Autodesk Fusion 360 part; units mm, degrees
(part 4 of 5)
sketch "Sketch4" plane through (0, 0, 0) normal (0, 0, -1) x (-1, 0, 0)
  arc A0 (-100, 198) -> (-100, 202) centre (-100, 200) ccw
  line L0 (-100, 198) -> (-100, 162)
  arc A1 (-100, 158) -> (-100, 162) centre (-100, 160) ccw
  line L1 (-100, 158) -> (-100, 122)
  arc A2 (-100, 118) -> (-100, 122) centre (-100, 120) ccw
  line L2 (-100, 118) -> (-100, 82)
  arc A3 (-100, 78) -> (-100, 82) centre (-100, 80) ccw
  line L3 (-100, 78) -> (-100, 42)
  arc A4 (-100, 38) -> (-100, 42) centre (-100, 40) ccw
  line L4 (-100, 38) -> (-100, 2)
  arc A5 (-100, -2) -> (-100, 2) centre (-100, 0) ccw
  line L5 (-100, -2) -> (-100, -38)
  arc A6 (-100, -42) -> (-100, -38) centre (-100, -40) ccw
  line L6 (-100, -42) -> (-100, -78)
  arc A7 (-100, -82) -> (-100, -78) centre (-100, -80) ccw
  line L7 (-100, -82) -> (-100, -118)
  arc A8 (-100, -122) -> (-100, -118) centre (-100, -120) ccw
  line L8 (-100, -122) -> (-100, -158)
  arc A9 (-100, -162) -> (-100, -158) centre (-100, -160) ccw
  line L9 (-100, -162) -> (-100, -198)
  arc A10 (-100, -202) -> (-100, -198) centre (-100, -200) ccw
  line L10 (-100, -202) -> (-100, -220)
  line L11 (-100, -220) -> (100, -220)
  line L12 (100, -220) -> (100, 220)
  line L13 (100, 220) -> (-100, 220)
  line L14 (-100, 220) -> (-100, 202)
  line L15 (38.5, 121.5) -> (21.5, 121.5)
  line L16 (21.5, 121.5) -> (21.5, 138.5)
  line L17 (21.5, 138.5) -> (38.5, 138.5)
  line L18 (38.5, 138.5) -> (38.5, 121.5)
  line L19 (18.5, 121.5) -> (1.5, 121.5)
  line L20 (1.5, 121.5) -> (1.5, 138.5)
  line L21 (1.5, 138.5) -> (18.5, 138.5)
  line L22 (18.5, 138.5) -> (18.5, 121.5)
  line L23 (-1.5, 121.5) -> (-18.5, 121.5)
  line L24 (-18.5, 121.5) -> (-18.5, 138.5)
  line L25 (-18.5, 138.5) -> (-1.5, 138.5)
  line L26 (-1.5, 138.5) -> (-1.5, 121.5)
  line L27 (-21.5, 121.5) -> (-38.5, 121.5)
  line L28 (-38.5, 121.5) -> (-38.5, 138.5)
  line L29 (-38.5, 138.5) -> (-21.5, 138.5)
  line L30 (-21.5, 138.5) -> (-21.5, 121.5)
  line L31 (-41.5, 121.5) -> (-58.5, 121.5)
  line L32 (-58.5, 121.5) -> (-58.5, 138.5)
  line L33 (-58.5, 138.5) -> (-41.5, 138.5)
  line L34 (-41.5, 138.5) -> (-41.5, 121.5)
  line L35 (-61.5, 121.5) -> (-78.5, 121.5)
  line L36 (-78.5, 121.5) -> (-78.5, 138.5)
  line L37 (-78.5, 138.5) -> (-61.5, 138.5)
  line L38 (-61.5, 138.5) -> (-61.5, 121.5)
  line L39 (-81.5, 121.5) -> (-98.5, 121.5)
  line L40 (-98.5, 121.5) -> (-98.5, 138.5)
  line L41 (-98.5, 138.5) -> (-81.5, 138.5)
  line L42 (-81.5, 138.5) -> (-81.5, 121.5)
  line L43 (98.5, 141.5) -> (81.5, 141.5)
  line L44 (81.5, 141.5) -> (81.5, 158.5)
  line L45 (81.5, 158.5) -> (98.5, 158.5)
  line L46 (98.5, 158.5) -> (98.5, 141.5)
  line L47 (78.5, 141.5) -> (61.5, 141.5)
  line L48 (61.5, 141.5) -> (61.5, 158.5)
  line L49 (61.5, 158.5) -> (78.5, 158.5)
  line L50 (78.5, 158.5) -> (78.5, 141.5)
  line L51 (58.5, 141.5) -> (41.5, 141.5)
  line L52 (41.5, 141.5) -> (41.5, 158.5)
  line L53 (41.5, 158.5) -> (58.5, 158.5)
  line L54 (58.5, 158.5) -> (58.5, 141.5)
  line L55 (38.5, 141.5) -> (21.5, 141.5)
  line L56 (21.5, 141.5) -> (21.5, 158.5)
  line L57 (21.5, 158.5) -> (38.5, 158.5)
  line L58 (38.5, 158.5) -> (38.5, 141.5)
  line L59 (18.5, 141.5) -> (1.5, 141.5)
  line L60 (1.5, 141.5) -> (1.5, 158.5)
  line L61 (1.5, 158.5) -> (18.5, 158.5)
  line L62 (18.5, 158.5) -> (18.5, 141.5)
  line L63 (-1.5, 141.5) -> (-18.5, 141.5)
  line L64 (-18.5, 141.5) -> (-18.5, 158.5)
  line L65 (-18.5, 158.5) -> (-1.5, 158.5)
  line L66 (-1.5, 158.5) -> (-1.5, 141.5)
  line L67 (-21.5, 141.5) -> (-38.5, 141.5)
  line L68 (-38.5, 141.5) -> (-38.5, 158.5)
  line L69 (-38.5, 158.5) -> (-21.5, 158.5)
  line L70 (-21.5, 158.5) -> (-21.5, 141.5)
  line L71 (-41.5, 141.5) -> (-58.5, 141.5)
  line L72 (-58.5, 141.5) -> (-58.5, 158.5)
  line L73 (-58.5, 158.5) -> (-41.5, 158.5)
  line L74 (-41.5, 158.5) -> (-41.5, 141.5)
  line L75 (-61.5, 141.5) -> (-78.5, 141.5)
  line L76 (-78.5, 141.5) -> (-78.5, 158.5)
  line L77 (-78.5, 158.5) -> (-61.5, 158.5)
  line L78 (-61.5, 158.5) -> (-61.5, 141.5)
  line L79 (-81.5, 141.5) -> (-98.5, 141.5)
  line L80 (-98.5, 141.5) -> (-98.5, 158.5)
  line L81 (-98.5, 158.5) -> (-81.5, 158.5)
  line L82 (-81.5, 158.5) -> (-81.5, 141.5)
  line L83 (98.5, 161.5) -> (81.5, 161.5)
  line L84 (81.5, 161.5) -> (81.5, 178.5)
  line L85 (81.5, 178.5) -> (98.5, 178.5)
  line L86 (98.5, 178.5) -> (98.5, 161.5)
  line L87 (78.5, 161.5) -> (61.5, 161.5)
  line L88 (61.5, 161.5) -> (61.5, 178.5)
  line L89 (61.5, 178.5) -> (78.5, 178.5)
  line L90 (78.5, 178.5) -> (78.5, 161.5)
  line L91 (58.5, 161.5) -> (41.5, 161.5)
  line L92 (41.5, 161.5) -> (41.5, 178.5)
  line L93 (41.5, 178.5) -> (58.5, 178.5)
  line L94 (58.5, 178.5) -> (58.5, 161.5)
  line L95 (58.5, 121.5) -> (41.5, 121.5)
  line L96 (41.5, 121.5) -> (41.5, 138.5)
  line L97 (41.5, 138.5) -> (58.5, 138.5)
  line L98 (58.5, 138.5) -> (58.5, 121.5)
  line L99 (98.5, -98.5) -> (81.5, -98.5)
  line L100 (81.5, -98.5) -> (81.5, -81.5)
  line L101 (81.5, -81.5) -> (98.5, -81.5)
  line L102 (98.5, -81.5) -> (98.5, -98.5)
  line L103 (-1.5, -58.5) -> (-18.5, -58.5)
  line L104 (-18.5, -58.5) -> (-18.5, -41.5)
  line L105 (-18.5, -41.5) -> (-1.5, -41.5)
  line L106 (-1.5, -41.5) -> (-1.5, -58.5)
  line L107 (-81.5, -118.5) -> (-98.5, -118.5)
  line L108 (-98.5, -118.5) -> (-98.5, -101.5)
  line L109 (-98.5, -101.5) -> (-81.5, -101.5)
  line L110 (-81.5, -101.5) -> (-81.5, -118.5)
  line L111 (-61.5, -118.5) -> (-78.5, -118.5)
  line L112 (-78.5, -118.5) -> (-78.5, -101.5)
  line L113 (-78.5, -101.5) -> (-61.5, -101.5)
  line L114 (-61.5, -101.5) -> (-61.5, -118.5)
  line L115 (-41.5, -118.5) -> (-58.5, -118.5)
  line L116 (-58.5, -118.5) -> (-58.5, -101.5)
  line L117 (-58.5, -101.5) -> (-41.5, -101.5)
  line L118 (-41.5, -101.5) -> (-41.5, -118.5)
  line L119 (-21.5, -118.5) -> (-38.5, -118.5)
  line L120 (-38.5, -118.5) -> (-38.5, -101.5)
  line L121 (-38.5, -101.5) -> (-21.5, -101.5)
  line L122 (-21.5, -101.5) -> (-21.5, -118.5)
  line L123 (-1.5, -118.5) -> (-18.5, -118.5)
  line L124 (-18.5, -118.5) -> (-18.5, -101.5)
  line L125 (-18.5, -101.5) -> (-1.5, -101.5)
  line L126 (-1.5, -101.5) -> (-1.5, -118.5)
  line L127 (18.5, -118.5) -> (1.5, -118.5)
  line L128 (1.5, -118.5) -> (1.5, -101.5)
  line L129 (1.5, -101.5) -> (18.5, -101.5)
  line L130 (18.5, -101.5) -> (18.5, -118.5)
  line L131 (38.5, -118.5) -> (21.5, -118.5)
  line L132 (21.5, -118.5) -> (21.5, -101.5)
  line L133 (21.5, -101.5) -> (38.5, -101.5)
  line L134 (38.5, -101.5) -> (38.5, -118.5)
  line L135 (58.5, -118.5) -> (41.5, -118.5)
  line L136 (41.5, -118.5) -> (41.5, -101.5)
  line L137 (41.5, -101.5) -> (58.5, -101.5)
  line L138 (58.5, -101.5) -> (58.5, -118.5)
  line L139 (78.5, -118.5) -> (61.5, -118.5)
  line L140 (61.5, -118.5) -> (61.5, -101.5)
  line L141 (61.5, -101.5) -> (78.5, -101.5)
  line L142 (78.5, -101.5) -> (78.5, -118.5)
  line L143 (98.5, -118.5) -> (81.5, -118.5)
  line L144 (81.5, -118.5) -> (81.5, -101.5)
  line L145 (81.5, -101.5) -> (98.5, -101.5)
  line L146 (98.5, -101.5) -> (98.5, -118.5)
  line L147 (-81.5, -138.5) -> (-98.5, -138.5)
  line L148 (-98.5, -138.5) -> (-98.5, -121.5)
  line L149 (-98.5, -121.5) -> (-81.5, -121.5)
  line L150 (-81.5, -121.5) -> (-81.5, -138.5)
  line L151 (-61.5, -138.5) -> (-78.5, -138.5)
  line L152 (-78.5, -138.5) -> (-78.5, -121.5)
  line L153 (-78.5, -121.5) -> (-61.5, -121.5)
  line L154 (-61.5, -121.5) -> (-61.5, -138.5)
  line L155 (-41.5, -138.5) -> (-58.5, -138.5)
  line L156 (-58.5, -138.5) -> (-58.5, -121.5)
  line L157 (-58.5, -121.5) -> (-41.5, -121.5)
  line L158 (-41.5, -121.5) -> (-41.5, -138.5)
  line L159 (-21.5, -138.5) -> (-38.5, -138.5)
  line L160 (-38.5, -138.5) -> (-38.5, -121.5)
  line L161 (-38.5, -121.5) -> (-21.5, -121.5)
  line L162 (-21.5, -121.5) -> (-21.5, -138.5)
  line L163 (-1.5, -138.5) -> (-18.5, -138.5)
  line L164 (-18.5, -138.5) -> (-18.5, -121.5)
  line L165 (-18.5, -121.5) -> (-1.5, -121.5)
  line L166 (-1.5, -121.5) -> (-1.5, -138.5)
  line L167 (18.5, -138.5) -> (1.5, -138.5)
  line L168 (1.5, -138.5) -> (1.5, -121.5)
  line L169 (1.5, -121.5) -> (18.5, -121.5)
  line L170 (18.5, -121.5) -> (18.5, -138.5)
  line L171 (38.5, -138.5) -> (21.5, -138.5)
  line L172 (21.5, -138.5) -> (21.5, -121.5)
  line L173 (21.5, -121.5) -> (38.5, -121.5)
  line L174 (38.5, -121.5) -> (38.5, -138.5)
  line L175 (58.5, -138.5) -> (41.5, -138.5)
  line L176 (41.5, -138.5) -> (41.5, -121.5)
  line L177 (41.5, -121.5) -> (58.5, -121.5)
  line L178 (58.5, -121.5) -> (58.5, -138.5)
  line L179 (78.5, -138.5) -> (61.5, -138.5)
  line L180 (61.5, -138.5) -> (61.5, -121.5)
  line L181 (61.5, -121.5) -> (78.5, -121.5)
  line L182 (78.5, -121.5) -> (78.5, -138.5)
  line L183 (98.5, -138.5) -> (81.5, -138.5)
  line L184 (81.5, -138.5) -> (81.5, -121.5)
  line L185 (81.5, -121.5) -> (98.5, -121.5)
  line L186 (98.5, -121.5) -> (98.5, -138.5)
  line L187 (-81.5, -158.5) -> (-98.5, -158.5)
  line L188 (-98.5, -158.5) -> (-98.5, -141.5)
  line L189 (-98.5, -141.5) -> (-81.5, -141.5)
  line L190 (-81.5, -141.5) -> (-81.5, -158.5)
  line L191 (-61.5, -158.5) -> (-78.5, -158.5)
  line L192 (-78.5, -158.5) -> (-78.5, -141.5)
  line L193 (-78.5, -141.5) -> (-61.5, -141.5)
  line L194 (-61.5, -141.5) -> (-61.5, -158.5)
  line L195 (-41.5, -158.5) -> (-58.5, -158.5)
  line L196 (-58.5, -158.5) -> (-58.5, -141.5)
  line L197 (-58.5, -141.5) -> (-41.5, -141.5)
  line L198 (-41.5, -141.5) -> (-41.5, -158.5)
  line L199 (-21.5, -158.5) -> (-38.5, -158.5)
  line L200 (-38.5, -158.5) -> (-38.5, -141.5)
  line L201 (-38.5, -141.5) -> (-21.5, -141.5)
  line L202 (-21.5, -141.5) -> (-21.5, -158.5)
  line L203 (-1.5, -158.5) -> (-18.5, -158.5)
  line L204 (-18.5, -158.5) -> (-18.5, -141.5)
  line L205 (-18.5, -141.5) -> (-1.5, -141.5)
  line L206 (-1.5, -141.5) -> (-1.5, -158.5)
  line L207 (18.5, -158.5) -> (1.5, -158.5)
  line L208 (1.5, -158.5) -> (1.5, -141.5)
  line L209 (1.5, -141.5) -> (18.5, -141.5)
  line L210 (18.5, -141.5) -> (18.5, -158.5)
  line L211 (38.5, -158.5) -> (21.5, -158.5)
  line L212 (21.5, -158.5) -> (21.5, -141.5)
  line L213 (21.5, -141.5) -> (38.5, -141.5)
  line L214 (38.5, -141.5) -> (38.5, -158.5)
  line L215 (58.5, -158.5) -> (41.5, -158.5)
  line L216 (41.5, -158.5) -> (41.5, -141.5)
  line L217 (41.5, -141.5) -> (58.5, -141.5)
  line L218 (58.5, -141.5) -> (58.5, -158.5)
  line L219 (-41.5, -58.5) -> (-58.5, -58.5)
  line L220 (-58.5, -58.5) -> (-58.5, -41.5)
  line L221 (-58.5, -41.5) -> (-41.5, -41.5)
  line L222 (-41.5, -41.5) -> (-41.5, -58.5)
  line L223 (98.5, -201.5) -> (98.5, -218.5)
  line L224 (98.5, -218.5) -> (81.5, -218.5)
  line L225 (81.5, -218.5) -> (81.5, -201.5)
  line L226 (81.5, -201.5) -> (98.5, -201.5)
  line L227 (78.5, -218.5) -> (61.5, -218.5)
  line L228 (61.5, -218.5) -> (61.5, -201.5)
  line L229 (61.5, -201.5) -> (78.5, -201.5)
  line L230 (78.5, -201.5) -> (78.5, -218.5)
  line L231 (58.5, -218.5) -> (41.5, -218.5)
  line L232 (41.5, -218.5) -> (41.5, -201.5)
  line L233 (41.5, -201.5) -> (58.5, -201.5)
  line L234 (58.5, -201.5) -> (58.5, -218.5)
  line L235 (38.5, -218.5) -> (21.5, -218.5)
  line L236 (21.5, -218.5) -> (21.5, -201.5)
  line L237 (21.5, -201.5) -> (38.5, -201.5)
  line L238 (38.5, -201.5) -> (38.5, -218.5)
  line L239 (18.5, -218.5) -> (1.5, -218.5)
  line L240 (1.5, -218.5) -> (1.5, -201.5)
  line L241 (1.5, -201.5) -> (18.5, -201.5)
  line L242 (18.5, -201.5) -> (18.5, -218.5)
  line L243 (-1.5, -218.5) -> (-18.5, -218.5)
  line L244 (-18.5, -218.5) -> (-18.5, -201.5)
  line L245 (-18.5, -201.5) -> (-1.5, -201.5)
  line L246 (-1.5, -201.5) -> (-1.5, -218.5)
  line L247 (-21.5, -218.5) -> (-38.5, -218.5)
  line L248 (-38.5, -218.5) -> (-38.5, -201.5)
  line L249 (-38.5, -201.5) -> (-21.5, -201.5)
  line L250 (-21.5, -201.5) -> (-21.5, -218.5)
  line L251 (-41.5, -218.5) -> (-58.5, -218.5)
  line L252 (-58.5, -218.5) -> (-58.5, -201.5)
  line L253 (-58.5, -201.5) -> (-41.5, -201.5)
  line L254 (-41.5, -201.5) -> (-41.5, -218.5)
  line L255 (-61.5, -218.5) -> (-78.5, -218.5)
  line L256 (-78.5, -218.5) -> (-78.5, -201.5)
  line L257 (-78.5, -201.5) -> (-61.5, -201.5)
  line L258 (-61.5, -201.5) -> (-61.5, -218.5)
  line L259 (-81.5, -218.5) -> (-98.5, -218.5)
  line L260 (-98.5, -218.5) -> (-98.5, -201.5)
  line L261 (-98.5, -201.5) -> (-81.5, -201.5)
  line L262 (-81.5, -201.5) -> (-81.5, -218.5)
  line L263 (98.5, -198.5) -> (81.5, -198.5)
  line L264 (81.5, -198.5) -> (81.5, -181.5)
  line L265 (81.5, -181.5) -> (98.5, -181.5)
  line L266 (98.5, -181.5) -> (98.5, -198.5)
  line L267 (78.5, -198.5) -> (61.5, -198.5)
  line L268 (61.5, -198.5) -> (61.5, -181.5)
  line L269 (61.5, -181.5) -> (78.5, -181.5)
  line L270 (78.5, -181.5) -> (78.5, -198.5)
  line L271 (58.5, -198.5) -> (41.5, -198.5)
  line L272 (41.5, -198.5) -> (41.5, -181.5)
  line L273 (41.5, -181.5) -> (58.5, -181.5)
  line L274 (58.5, -181.5) -> (58.5, -198.5)
  line L275 (38.5, -198.5) -> (21.5, -198.5)
  line L276 (21.5, -198.5) -> (21.5, -181.5)
  line L277 (21.5, -181.5) -> (38.5, -181.5)
  line L278 (38.5, -181.5) -> (38.5, -198.5)
  line L279 (18.5, -198.5) -> (1.5, -198.5)
  line L280 (1.5, -198.5) -> (1.5, -181.5)
  line L281 (1.5, -181.5) -> (18.5, -181.5)
  line L282 (18.5, -181.5) -> (18.5, -198.5)
  line L283 (-1.5, -198.5) -> (-18.5, -198.5)
  line L284 (-18.5, -198.5) -> (-18.5, -181.5)
  line L285 (-18.5, -181.5) -> (-1.5, -181.5)
  line L286 (-1.5, -181.5) -> (-1.5, -198.5)
  line L287 (-21.5, -198.5) -> (-38.5, -198.5)
  line L288 (-38.5, -198.5) -> (-38.5, -181.5)
  line L289 (-38.5, -181.5) -> (-21.5, -181.5)
  line L290 (-21.5, -181.5) -> (-21.5, -198.5)
  line L291 (-41.5, -198.5) -> (-58.5, -198.5)
  line L292 (-58.5, -198.5) -> (-58.5, -181.5)
  line L293 (-58.5, -181.5) -> (-41.5, -181.5)
  line L294 (-41.5, -181.5) -> (-41.5, -198.5)
  line L295 (-61.5, -198.5) -> (-78.5, -198.5)
  line L296 (-78.5, -198.5) -> (-78.5, -181.5)
  line L297 (-78.5, -181.5) -> (-61.5, -181.5)
  line L298 (-61.5, -181.5) -> (-61.5, -198.5)
  line L299 (-81.5, -198.5) -> (-98.5, -198.5)
  line L300 (-98.5, -198.5) -> (-98.5, -181.5)
  line L301 (-98.5, -181.5) -> (-81.5, -181.5)
  line L302 (-81.5, -181.5) -> (-81.5, -198.5)
  line L303 (98.5, -178.5) -> (81.5, -178.5)
  line L304 (81.5, -178.5) -> (81.5, -161.5)
  line L305 (81.5, -161.5) -> (98.5, -161.5)
  line L306 (98.5, -161.5) -> (98.5, -178.5)
  line L307 (78.5, -178.5) -> (61.5, -178.5)
  line L308 (61.5, -178.5) -> (61.5, -161.5)
  line L309 (61.5, -161.5) -> (78.5, -161.5)
  line L310 (78.5, -161.5) -> (78.5, -178.5)
  line L311 (58.5, -178.5) -> (41.5, -178.5)
  line L312 (41.5, -178.5) -> (41.5, -161.5)
  line L313 (41.5, -161.5) -> (58.5, -161.5)
  line L314 (58.5, -161.5) -> (58.5, -178.5)
  line L315 (38.5, -178.5) -> (21.5, -178.5)
  line L316 (21.5, -178.5) -> (21.5, -161.5)
  line L317 (21.5, -161.5) -> (38.5, -161.5)
  line L318 (38.5, -161.5) -> (38.5, -178.5)
  line L319 (18.5, -178.5) -> (1.5, -178.5)
  line L320 (1.5, -178.5) -> (1.5, -161.5)
  line L321 (1.5, -161.5) -> (18.5, -161.5)
  line L322 (18.5, -161.5) -> (18.5, -178.5)
  line L323 (-1.5, -178.5) -> (-18.5, -178.5)
  line L324 (-18.5, -178.5) -> (-18.5, -161.5)
  line L325 (-18.5, -161.5) -> (-1.5, -161.5)
  line L326 (-1.5, -161.5) -> (-1.5, -178.5)
  line L327 (98.5, -158.5) -> (81.5, -158.5)
  line L328 (81.5, -158.5) -> (81.5, -141.5)
  line L329 (81.5, -141.5) -> (98.5, -141.5)
  line L330 (98.5, -141.5) -> (98.5, -158.5)
  line L331 (78.5, -158.5) -> (61.5, -158.5)
  line L332 (61.5, -158.5) -> (61.5, -141.5)
  line L333 (61.5, -141.5) -> (78.5, -141.5)
  line L334 (78.5, -141.5) -> (78.5, -158.5)
  line L335 (-81.5, -178.5) -> (-98.5, -178.5)
  line L336 (-98.5, -178.5) -> (-98.5, -161.5)
  line L337 (-98.5, -161.5) -> (-81.5, -161.5)
  line L338 (-81.5, -161.5) -> (-81.5, -178.5)
  line L339 (-61.5, -178.5) -> (-78.5, -178.5)
  line L340 (-78.5, -178.5) -> (-78.5, -161.5)
  line L341 (-78.5, -161.5) -> (-61.5, -161.5)
  line L342 (-61.5, -161.5) -> (-61.5, -178.5)
  line L343 (-41.5, -178.5) -> (-58.5, -178.5)
  line L344 (-58.5, -178.5) -> (-58.5, -161.5)
  line L345 (-58.5, -161.5) -> (-41.5, -161.5)
  line L346 (-41.5, -161.5) -> (-41.5, -178.5)
  line L347 (-21.5, -178.5) -> (-38.5, -178.5)
  line L348 (-38.5, -178.5) -> (-38.5, -161.5)
  line L349 (-38.5, -161.5) -> (-21.5, -161.5)
  line L350 (-21.5, -161.5) -> (-21.5, -178.5)
  line L351 (38.5, 161.5) -> (21.5, 161.5)
  line L352 (21.5, 161.5) -> (21.5, 178.5)
  line L353 (21.5, 178.5) -> (38.5, 178.5)
  line L354 (38.5, 178.5) -> (38.5, 161.5)
  line L355 (78.5, -98.5) -> (61.5, -98.5)
  line L356 (61.5, -98.5) -> (61.5, -81.5)
  line L357 (61.5, -81.5) -> (78.5, -81.5)
  line L358 (78.5, -81.5) -> (78.5, -98.5)
  line L359 (98.5, 121.5) -> (81.5, 121.5)
  line L360 (81.5, 121.5) -> (81.5, 138.5)
  line L361 (81.5, 138.5) -> (98.5, 138.5)
  line L362 (98.5, 138.5) -> (98.5, 121.5)
  line L363 (-81.5, 101.5) -> (-98.5, 101.5)
  line L364 (-98.5, 101.5) -> (-98.5, 118.5)
  line L365 (-98.5, 118.5) -> (-81.5, 118.5)
  line L366 (-81.5, 118.5) -> (-81.5, 101.5)
  line L367 (-61.5, 101.5) -> (-78.5, 101.5)
  line L368 (-78.5, 101.5) -> (-78.5, 118.5)
  line L369 (-78.5, 118.5) -> (-61.5, 118.5)
  line L370 (-61.5, 118.5) -> (-61.5, 101.5)
  line L371 (-41.5, 101.5) -> (-58.5, 101.5)
  line L372 (-58.5, 101.5) -> (-58.5, 118.5)
  line L373 (-58.5, 118.5) -> (-41.5, 118.5)
  line L374 (-41.5, 118.5) -> (-41.5, 101.5)
  line L375 (-21.5, 101.5) -> (-38.5, 101.5)
  line L376 (-38.5, 101.5) -> (-38.5, 118.5)
  line L377 (-38.5, 118.5) -> (-21.5, 118.5)
  line L378 (-21.5, 118.5) -> (-21.5, 101.5)
  line L379 (-1.5, 101.5) -> (-18.5, 101.5)
  line L380 (-18.5, 101.5) -> (-18.5, 118.5)
  line L381 (-18.5, 118.5) -> (-1.5, 118.5)
  line L382 (-1.5, 118.5) -> (-1.5, 101.5)
  line L383 (18.5, 101.5) -> (1.5, 101.5)
  line L384 (1.5, 101.5) -> (1.5, 118.5)
  line L385 (1.5, 118.5) -> (18.5, 118.5)
  line L386 (18.5, 118.5) -> (18.5, 101.5)
  line L387 (38.5, 101.5) -> (21.5, 101.5)
  line L388 (21.5, 101.5) -> (21.5, 118.5)
  line L389 (21.5, 118.5) -> (38.5, 118.5)
  line L390 (38.5, 118.5) -> (38.5, 101.5)
  line L391 (58.5, 101.5) -> (41.5, 101.5)
  line L392 (41.5, 101.5) -> (41.5, 118.5)
  line L393 (41.5, 118.5) -> (58.5, 118.5)
  line L394 (58.5, 118.5) -> (58.5, 101.5)
  line L395 (78.5, 101.5) -> (61.5, 101.5)
  line L396 (61.5, 101.5) -> (61.5, 118.5)
  line L397 (61.5, 118.5) -> (78.5, 118.5)
  line L398 (78.5, 118.5) -> (78.5, 101.5)
  line L399 (98.5, 101.5) -> (81.5, 101.5)
  line L400 (81.5, 101.5) -> (81.5, 118.5)
  line L401 (81.5, 118.5) -> (98.5, 118.5)
  line L402 (98.5, 118.5) -> (98.5, 101.5)
  line L403 (-81.5, 81.5) -> (-98.5, 81.5)
  line L404 (-98.5, 81.5) -> (-98.5, 98.5)
  line L405 (-98.5, 98.5) -> (-81.5, 98.5)
  line L406 (-81.5, 98.5) -> (-81.5, 81.5)
  line L407 (-61.5, 81.5) -> (-78.5, 81.5)
  line L408 (-78.5, 81.5) -> (-78.5, 98.5)
  line L409 (-78.5, 98.5) -> (-61.5, 98.5)
  line L410 (-61.5, 98.5) -> (-61.5, 81.5)
  line L411 (-41.5, 81.5) -> (-58.5, 81.5)
  line L412 (-58.5, 81.5) -> (-58.5, 98.5)
  line L413 (-58.5, 98.5) -> (-41.5, 98.5)
  line L414 (-41.5, 98.5) -> (-41.5, 81.5)
  line L415 (-21.5, 81.5) -> (-38.5, 81.5)
  line L416 (-38.5, 81.5) -> (-38.5, 98.5)
  line L417 (-38.5, 98.5) -> (-21.5, 98.5)
  line L418 (-21.5, 98.5) -> (-21.5, 81.5)
  line L419 (-1.5, 81.5) -> (-18.5, 81.5)
  line L420 (-18.5, 81.5) -> (-18.5, 98.5)
  line L421 (-18.5, 98.5) -> (-1.5, 98.5)
  line L422 (-1.5, 98.5) -> (-1.5, 81.5)
  line L423 (18.5, 81.5) -> (1.5, 81.5)
  line L424 (1.5, 81.5) -> (1.5, 98.5)
  line L425 (1.5, 98.5) -> (18.5, 98.5)
  line L426 (18.5, 98.5) -> (18.5, 81.5)
  line L427 (38.5, 81.5) -> (21.5, 81.5)
  line L428 (21.5, 81.5) -> (21.5, 98.5)
  line L429 (21.5, 98.5) -> (38.5, 98.5)
  line L430 (38.5, 98.5) -> (38.5, 81.5)
  line L431 (58.5, 81.5) -> (41.5, 81.5)
  line L432 (41.5, 81.5) -> (41.5, 98.5)
  line L433 (41.5, 98.5) -> (58.5, 98.5)
  line L434 (58.5, 98.5) -> (58.5, 81.5)
  line L435 (78.5, 81.5) -> (61.5, 81.5)
  line L436 (61.5, 81.5) -> (61.5, 98.5)
  line L437 (61.5, 98.5) -> (78.5, 98.5)
  line L438 (78.5, 98.5) -> (78.5, 81.5)
  line L439 (98.5, 81.5) -> (81.5, 81.5)
  line L440 (81.5, 81.5) -> (81.5, 98.5)
  line L441 (81.5, 98.5) -> (98.5, 98.5)
  line L442 (98.5, 98.5) -> (98.5, 81.5)
  line L443 (-81.5, 61.5) -> (-98.5, 61.5)
  line L444 (-98.5, 61.5) -> (-98.5, 78.5)
  line L445 (-98.5, 78.5) -> (-81.5, 78.5)
  line L446 (-81.5, 78.5) -> (-81.5, 61.5)
  line L447 (-61.5, 61.5) -> (-78.5, 61.5)
  line L448 (-78.5, 61.5) -> (-78.5, 78.5)
  line L449 (-78.5, 78.5) -> (-61.5, 78.5)
  line L450 (-61.5, 78.5) -> (-61.5, 61.5)
  line L451 (-41.5, 61.5) -> (-58.5, 61.5)
  line L452 (-58.5, 61.5) -> (-58.5, 78.5)
  line L453 (-58.5, 78.5) -> (-41.5, 78.5)
  line L454 (-41.5, 78.5) -> (-41.5, 61.5)
  line L455 (-21.5, 61.5) -> (-38.5, 61.5)
  line L456 (-38.5, 61.5) -> (-38.5, 78.5)
  line L457 (-38.5, 78.5) -> (-21.5, 78.5)
  line L458 (-21.5, 78.5) -> (-21.5, 61.5)
  line L459 (-1.5, 61.5) -> (-18.5, 61.5)
  line L460 (-18.5, 61.5) -> (-18.5, 78.5)
  line L461 (-18.5, 78.5) -> (-1.5, 78.5)
  line L462 (-1.5, 78.5) -> (-1.5, 61.5)
  line L463 (18.5, 61.5) -> (1.5, 61.5)
  line L464 (1.5, 61.5) -> (1.5, 78.5)
  line L465 (1.5, 78.5) -> (18.5, 78.5)
  line L466 (18.5, 78.5) -> (18.5, 61.5)
  line L467 (38.5, 61.5) -> (21.5, 61.5)
  line L468 (21.5, 61.5) -> (21.5, 78.5)
  line L469 (21.5, 78.5) -> (38.5, 78.5)
  line L470 (38.5, 78.5) -> (38.5, 61.5)
  line L471 (58.5, 61.5) -> (41.5, 61.5)
  line L472 (41.5, 61.5) -> (41.5, 78.5)
  line L473 (41.5, 78.5) -> (58.5, 78.5)
  line L474 (58.5, 78.5) -> (58.5, 61.5)
  line L475 (78.5, 61.5) -> (61.5, 61.5)
  line L476 (61.5, 61.5) -> (61.5, 78.5)
  line L477 (61.5, 78.5) -> (78.5, 78.5)
  line L478 (78.5, 78.5) -> (78.5, 61.5)
  line L479 (98.5, 61.5) -> (81.5, 61.5)
  line L480 (81.5, 61.5) -> (81.5, 78.5)
  line L481 (81.5, 78.5) -> (98.5, 78.5)
  line L482 (98.5, 78.5) -> (98.5, 61.5)
  line L483 (-81.5, 41.5) -> (-98.5, 41.5)
  line L484 (-98.5, 41.5) -> (-98.5, 58.5)
  line L485 (-98.5, 58.5) -> (-81.5, 58.5)
  line L486 (-81.5, 58.5) -> (-81.5, 41.5)
  line L487 (-61.5, 41.5) -> (-78.5, 41.5)
  line L488 (-78.5, 41.5) -> (-78.5, 58.5)
  line L489 (-78.5, 58.5) -> (-61.5, 58.5)
  line L490 (-61.5, 58.5) -> (-61.5, 41.5)
  line L491 (-41.5, 41.5) -> (-58.5, 41.5)
  line L492 (-58.5, 41.5) -> (-58.5, 58.5)
  line L493 (-58.5, 58.5) -> (-41.5, 58.5)
  line L494 (-41.5, 58.5) -> (-41.5, 41.5)
  line L495 (-21.5, 41.5) -> (-38.5, 41.5)
  line L496 (-38.5, 41.5) -> (-38.5, 58.5)
  line L497 (-38.5, 58.5) -> (-21.5, 58.5)
  line L498 (-21.5, 58.5) -> (-21.5, 41.5)
  line L499 (-1.5, 41.5) -> (-18.5, 41.5)
  line L500 (-18.5, 41.5) -> (-18.5, 58.5)
  line L501 (-18.5, 58.5) -> (-1.5, 58.5)
  line L502 (-1.5, 58.5) -> (-1.5, 41.5)
  line L503 (18.5, 41.5) -> (1.5, 41.5)
  line L504 (1.5, 41.5) -> (1.5, 58.5)
  line L505 (1.5, 58.5) -> (18.5, 58.5)
  line L506 (18.5, 58.5) -> (18.5, 41.5)
  line L507 (38.5, 41.5) -> (21.5, 41.5)
  line L508 (21.5, 41.5) -> (21.5, 58.5)
  line L509 (21.5, 58.5) -> (38.5, 58.5)
  line L510 (38.5, 58.5) -> (38.5, 41.5)
  line L511 (58.5, 41.5) -> (41.5, 41.5)
  line L512 (41.5, 41.5) -> (41.5, 58.5)
  line L513 (41.5, 58.5) -> (58.5, 58.5)
  line L514 (58.5, 58.5) -> (58.5, 41.5)
  line L515 (78.5, 41.5) -> (61.5, 41.5)
  line L516 (61.5, 41.5) -> (61.5, 58.5)
  line L517 (61.5, 58.5) -> (78.5, 58.5)
  line L518 (78.5, 58.5) -> (78.5, 41.5)
  line L519 (98.5, 41.5) -> (81.5, 41.5)
  line L520 (81.5, 41.5) -> (81.5, 58.5)
  line L521 (81.5, 58.5) -> (98.5, 58.5)
  line L522 (98.5, 58.5) -> (98.5, 41.5)
  line L523 (-81.5, 21.5) -> (-98.5, 21.5)
  line L524 (-98.5, 21.5) -> (-98.5, 38.5)
  line L525 (-98.5, 38.5) -> (-81.5, 38.5)
  line L526 (-81.5, 38.5) -> (-81.5, 21.5)
  line L527 (-61.5, 21.5) -> (-78.5, 21.5)
  line L528 (-78.5, 21.5) -> (-78.5, 38.5)
  line L529 (-78.5, 38.5) -> (-61.5, 38.5)
  line L530 (-61.5, 38.5) -> (-61.5, 21.5)
  line L531 (-41.5, 21.5) -> (-58.5, 21.5)
  line L532 (-58.5, 21.5) -> (-58.5, 38.5)
  line L533 (-58.5, 38.5) -> (-41.5, 38.5)
  line L534 (-41.5, 38.5) -> (-41.5, 21.5)
  line L535 (-21.5, 21.5) -> (-38.5, 21.5)
  line L536 (-38.5, 21.5) -> (-38.5, 38.5)
  line L537 (-38.5, 38.5) -> (-21.5, 38.5)
  line L538 (-21.5, 38.5) -> (-21.5, 21.5)
  line L539 (-1.5, 21.5) -> (-18.5, 21.5)
  line L540 (-18.5, 21.5) -> (-18.5, 38.5)
  line L541 (-18.5, 38.5) -> (-1.5, 38.5)
  line L542 (-1.5, 38.5) -> (-1.5, 21.5)
  line L543 (18.5, 21.5) -> (1.5, 21.5)
  line L544 (1.5, 21.5) -> (1.5, 38.5)
  line L545 (1.5, 38.5) -> (18.5, 38.5)
  line L546 (18.5, 38.5) -> (18.5, 21.5)
  line L547 (38.5, 21.5) -> (21.5, 21.5)
  line L548 (21.5, 21.5) -> (21.5, 38.5)
  line L549 (21.5, 38.5) -> (38.5, 38.5)
  line L550 (38.5, 38.5) -> (38.5, 21.5)
  line L551 (58.5, 21.5) -> (41.5, 21.5)
  line L552 (41.5, 21.5) -> (41.5, 38.5)
  line L553 (41.5, 38.5) -> (58.5, 38.5)
  line L554 (58.5, 38.5) -> (58.5, 21.5)
  line L555 (78.5, 21.5) -> (61.5, 21.5)
  line L556 (61.5, 21.5) -> (61.5, 38.5)
  line L557 (61.5, 38.5) -> (78.5, 38.5)
  line L558 (78.5, 38.5) -> (78.5, 21.5)
  line L559 (98.5, 21.5) -> (81.5, 21.5)
  line L560 (81.5, 21.5) -> (81.5, 38.5)
  line L561 (81.5, 38.5) -> (98.5, 38.5)
  line L562 (98.5, 38.5) -> (98.5, 21.5)
  line L563 (-81.5, 1.5) -> (-98.5, 1.5)
  line L564 (-98.5, 1.5) -> (-98.5, 18.5)
  line L565 (-98.5, 18.5) -> (-81.5, 18.5)
  line L566 (-81.5, 18.5) -> (-81.5, 1.5)
  line L567 (-61.5, 1.5) -> (-78.5, 1.5)
  line L568 (-78.5, 1.5) -> (-78.5, 18.5)
  line L569 (-78.5, 18.5) -> (-61.5, 18.5)
  line L570 (-61.5, 18.5) -> (-61.5, 1.5)
  line L571 (-41.5, 1.5) -> (-58.5, 1.5)
  line L572 (-58.5, 1.5) -> (-58.5, 18.5)
  line L573 (-58.5, 18.5) -> (-41.5, 18.5)
  line L574 (-41.5, 18.5) -> (-41.5, 1.5)
  line L575 (-21.5, 1.5) -> (-38.5, 1.5)
  line L576 (-38.5, 1.5) -> (-38.5, 18.5)
  line L577 (-38.5, 18.5) -> (-21.5, 18.5)
  line L578 (-21.5, 18.5) -> (-21.5, 1.5)
  line L579 (-1.5, 1.5) -> (-18.5, 1.5)
  line L580 (-18.5, 1.5) -> (-18.5, 18.5)
  line L581 (-18.5, 18.5) -> (-1.5, 18.5)
  line L582 (-1.5, 18.5) -> (-1.5, 1.5)
  line L583 (18.5, 1.5) -> (1.5, 1.5)
  line L584 (1.5, 1.5) -> (1.5, 18.5)
  line L585 (1.5, 18.5) -> (18.5, 18.5)
  line L586 (18.5, 18.5) -> (18.5, 1.5)
  line L587 (38.5, 1.5) -> (21.5, 1.5)
  line L588 (21.5, 1.5) -> (21.5, 18.5)
  line L589 (21.5, 18.5) -> (38.5, 18.5)
  line L590 (38.5, 18.5) -> (38.5, 1.5)
  line L591 (58.5, 1.5) -> (41.5, 1.5)
  line L592 (41.5, 1.5) -> (41.5, 18.5)
  line L593 (41.5, 18.5) -> (58.5, 18.5)
  line L594 (58.5, 18.5) -> (58.5, 1.5)
  line L595 (78.5, 1.5) -> (61.5, 1.5)
  line L596 (61.5, 1.5) -> (61.5, 18.5)
  line L597 (61.5, 18.5) -> (78.5, 18.5)
  line L598 (78.5, 18.5) -> (78.5, 1.5)
  line L599 (98.5, 1.5) -> (81.5, 1.5)
  line L600 (81.5, 1.5) -> (81.5, 18.5)
  line L601 (81.5, 18.5) -> (98.5, 18.5)
  line L602 (98.5, 18.5) -> (98.5, 1.5)
  line L603 (-81.5, -18.5) -> (-98.5, -18.5)
  line L604 (-98.5, -18.5) -> (-98.5, -1.5)
  line L605 (-98.5, -1.5) -> (-81.5, -1.5)
  line L606 (-81.5, -1.5) -> (-81.5, -18.5)
  line L607 (-61.5, -18.5) -> (-78.5, -18.5)
  line L608 (-78.5, -18.5) -> (-78.5, -1.5)
  line L609 (-78.5, -1.5) -> (-61.5, -1.5)
  line L610 (-61.5, -1.5) -> (-61.5, -18.5)
  line L611 (-41.5, -18.5) -> (-58.5, -18.5)
  line L612 (-58.5, -18.5) -> (-58.5, -1.5)
  line L613 (-58.5, -1.5) -> (-41.5, -1.5)
  line L614 (-41.5, -1.5) -> (-41.5, -18.5)
  line L615 (-21.5, -18.5) -> (-38.5, -18.5)
  line L616 (-38.5, -18.5) -> (-38.5, -1.5)
  line L617 (-38.5, -1.5) -> (-21.5, -1.5)
  line L618 (-21.5, -1.5) -> (-21.5, -18.5)
  line L619 (-1.5, -18.5) -> (-18.5, -18.5)
  line L620 (-18.5, -18.5) -> (-18.5, -1.5)
  line L621 (-18.5, -1.5) -> (-1.5, -1.5)
  line L622 (-1.5, -1.5) -> (-1.5, -18.5)
  line L623 (18.5, -18.5) -> (1.5, -18.5)
  line L624 (1.5, -18.5) -> (1.5, -1.5)
  line L625 (1.5, -1.5) -> (18.5, -1.5)
  line L626 (18.5, -1.5) -> (18.5, -18.5)
  line L627 (38.5, -18.5) -> (21.5, -18.5)
  line L628 (21.5, -18.5) -> (21.5, -1.5)
  line L629 (21.5, -1.5) -> (38.5, -1.5)
  line L630 (38.5, -1.5) -> (38.5, -18.5)
  line L631 (58.5, -18.5) -> (41.5, -18.5)
  line L632 (41.5, -18.5) -> (41.5, -1.5)
  line L633 (41.5, -1.5) -> (58.5, -1.5)
  line L634 (58.5, -1.5) -> (58.5, -18.5)
  line L635 (78.5, -18.5) -> (61.5, -18.5)
  line L636 (61.5, -18.5) -> (61.5, -1.5)
  line L637 (61.5, -1.5) -> (78.5, -1.5)
  line L638 (78.5, -1.5) -> (78.5, -18.5)
  line L639 (98.5, -18.5) -> (81.5, -18.5)
  line L640 (81.5, -18.5) -> (81.5, -1.5)
  line L641 (81.5, -1.5) -> (98.5, -1.5)
  line L642 (98.5, -1.5) -> (98.5, -18.5)
  line L643 (-81.5, -38.5) -> (-98.5, -38.5)
  line L644 (-98.5, -38.5) -> (-98.5, -21.5)
  line L645 (-98.5, -21.5) -> (-81.5, -21.5)
  line L646 (-81.5, -21.5) -> (-81.5, -38.5)
  line L647 (-61.5, -38.5) -> (-78.5, -38.5)
  line L648 (-78.5, -38.5) -> (-78.5, -21.5)
  line L649 (-78.5, -21.5) -> (-61.5, -21.5)
  line L650 (-61.5, -21.5) -> (-61.5, -38.5)
  line L651 (-41.5, -38.5) -> (-58.5, -38.5)
  line L652 (-58.5, -38.5) -> (-58.5, -21.5)
  line L653 (-58.5, -21.5) -> (-41.5, -21.5)
  line L654 (-41.5, -21.5) -> (-41.5, -38.5)
  line L655 (-21.5, -38.5) -> (-38.5, -38.5)
  line L656 (-38.5, -38.5) -> (-38.5, -21.5)
  line L657 (-38.5, -21.5) -> (-21.5, -21.5)
  line L658 (-21.5, -21.5) -> (-21.5, -38.5)
  line L659 (-1.5, -38.5) -> (-18.5, -38.5)
  line L660 (-18.5, -38.5) -> (-18.5, -21.5)
  line L661 (-18.5, -21.5) -> (-1.5, -21.5)
  line L662 (-1.5, -21.5) -> (-1.5, -38.5)
  line L663 (18.5, -38.5) -> (1.5, -38.5)
  line L664 (1.5, -38.5) -> (1.5, -21.5)
  line L665 (1.5, -21.5) -> (18.5, -21.5)
  line L666 (18.5, -21.5) -> (18.5, -38.5)
  line L667 (38.5, -38.5) -> (21.5, -38.5)
  line L668 (21.5, -38.5) -> (21.5, -21.5)
  line L669 (21.5, -21.5) -> (38.5, -21.5)
  line L670 (38.5, -21.5) -> (38.5, -38.5)
  line L671 (58.5, -38.5) -> (41.5, -38.5)
  line L672 (41.5, -38.5) -> (41.5, -21.5)
  line L673 (41.5, -21.5) -> (58.5, -21.5)
  line L674 (58.5, -21.5) -> (58.5, -38.5)
  line L675 (78.5, -38.5) -> (61.5, -38.5)
  line L676 (61.5, -38.5) -> (61.5, -21.5)
  line L677 (61.5, -21.5) -> (78.5, -21.5)
  line L678 (78.5, -21.5) -> (78.5, -38.5)
  line L679 (98.5, -38.5) -> (81.5, -38.5)
  line L680 (81.5, -38.5) -> (81.5, -21.5)
  line L681 (81.5, -21.5) -> (98.5, -21.5)
  line L682 (98.5, -21.5) -> (98.5, -38.5)
  line L683 (-81.5, -58.5) -> (-98.5, -58.5)
  line L684 (-98.5, -58.5) -> (-98.5, -41.5)
  line L685 (-98.5, -41.5) -> (-81.5, -41.5)
  line L686 (-81.5, -41.5) -> (-81.5, -58.5)
  line L687 (-61.5, -58.5) -> (-78.5, -58.5)
  line L688 (-78.5, -58.5) -> (-78.5, -41.5)
  line L689 (-78.5, -41.5) -> (-61.5, -41.5)
  line L690 (-61.5, -41.5) -> (-61.5, -58.5)
  line L691 (-81.5, 201.5) -> (-98.5, 201.5)
  line L692 (-98.5, 201.5) -> (-98.5, 218.5)
  line L693 (-98.5, 218.5) -> (-81.5, 218.5)
  line L694 (-81.5, 218.5) -> (-81.5, 201.5)
  line L695 (-61.5, 201.5) -> (-78.5, 201.5)
  line L696 (-78.5, 201.5) -> (-78.5, 218.5)
  line L697 (-78.5, 218.5) -> (-61.5, 218.5)
  line L698 (-61.5, 218.5) -> (-61.5, 201.5)
  line L699 (-41.5, 201.5) -> (-58.5, 201.5)
  line L700 (-58.5, 201.5) -> (-58.5, 218.5)
  line L701 (-58.5, 218.5) -> (-41.5, 218.5)
  line L702 (-41.5, 218.5) -> (-41.5, 201.5)
  line L703 (-21.5, 201.5) -> (-38.5, 201.5)
  line L704 (-38.5, 201.5) -> (-38.5, 218.5)
  line L705 (-38.5, 218.5) -> (-21.5, 218.5)
  line L706 (-21.5, 218.5) -> (-21.5, 201.5)
  line L707 (-1.5, 201.5) -> (-18.5, 201.5)
  line L708 (-18.5, 201.5) -> (-18.5, 218.5)
  line L709 (-18.5, 218.5) -> (-1.5, 218.5)
  line L710 (-1.5, 218.5) -> (-1.5, 201.5)
  line L711 (18.5, 201.5) -> (1.5, 201.5)
  line L712 (1.5, 201.5) -> (1.5, 218.5)
  line L713 (1.5, 218.5) -> (18.5, 218.5)
  line L714 (18.5, 218.5) -> (18.5, 201.5)
  line L715 (38.5, 201.5) -> (21.5, 201.5)
  line L716 (21.5, 201.5) -> (21.5, 218.5)
  line L717 (21.5, 218.5) -> (38.5, 218.5)
  line L718 (38.5, 218.5) -> (38.5, 201.5)
  line L719 (58.5, 201.5) -> (41.5, 201.5)
  line L720 (41.5, 201.5) -> (41.5, 218.5)
  line L721 (41.5, 218.5) -> (58.5, 218.5)
  line L722 (58.5, 218.5) -> (58.5, 201.5)
  line L723 (78.5, 201.5) -> (61.5, 201.5)
  line L724 (61.5, 201.5) -> (61.5, 218.5)
  line L725 (61.5, 218.5) -> (78.5, 218.5)
  line L726 (78.5, 218.5) -> (78.5, 201.5)
  line L727 (98.5, 201.5) -> (81.5, 201.5)
  line L728 (81.5, 201.5) -> (81.5, 218.5)
  line L729 (81.5, 218.5) -> (98.5, 218.5)
  line L730 (98.5, 218.5) -> (98.5, 201.5)
  line L731 (-81.5, 181.5) -> (-98.5, 181.5)
  line L732 (-98.5, 181.5) -> (-98.5, 198.5)
  line L733 (-98.5, 198.5) -> (-81.5, 198.5)
  line L734 (-81.5, 198.5) -> (-81.5, 181.5)
  line L735 (-61.5, 181.5) -> (-78.5, 181.5)
  line L736 (-78.5, 181.5) -> (-78.5, 198.5)
  line L737 (-78.5, 198.5) -> (-61.5, 198.5)
  line L738 (-61.5, 198.5) -> (-61.5, 181.5)
  line L739 (-41.5, 181.5) -> (-58.5, 181.5)
  line L740 (-58.5, 181.5) -> (-58.5, 198.5)
  line L741 (-58.5, 198.5) -> (-41.5, 198.5)
  line L742 (-41.5, 198.5) -> (-41.5, 181.5)
  line L743 (-21.5, 181.5) -> (-38.5, 181.5)
  line L744 (-38.5, 181.5) -> (-38.5, 198.5)
  line L745 (-38.5, 198.5) -> (-21.5, 198.5)
  line L746 (-21.5, 198.5) -> (-21.5, 181.5)
  line L747 (-1.5, 181.5) -> (-18.5, 181.5)
  line L748 (-18.5, 181.5) -> (-18.5, 198.5)
  line L749 (-18.5, 198.5) -> (-1.5, 198.5)
  line L750 (-1.5, 198.5) -> (-1.5, 181.5)
  line L751 (18.5, 181.5) -> (1.5, 181.5)
  line L752 (1.5, 181.5) -> (1.5, 198.5)
  line L753 (1.5, 198.5) -> (18.5, 198.5)
  line L754 (18.5, 198.5) -> (18.5, 181.5)
  line L755 (38.5, 181.5) -> (21.5, 181.5)
  line L756 (21.5, 181.5) -> (21.5, 198.5)
  line L757 (21.5, 198.5) -> (38.5, 198.5)
  line L758 (38.5, 198.5) -> (38.5, 181.5)
  line L759 (58.5, 181.5) -> (41.5, 181.5)
  line L760 (41.5, 181.5) -> (41.5, 198.5)
  line L761 (41.5, 198.5) -> (58.5, 198.5)
  line L762 (58.5, 198.5) -> (58.5, 181.5)
  line L763 (78.5, 181.5) -> (61.5, 181.5)
  line L764 (61.5, 181.5) -> (61.5, 198.5)
  line L765 (61.5, 198.5) -> (78.5, 198.5)
  line L766 (78.5, 198.5) -> (78.5, 181.5)
  line L767 (98.5, 181.5) -> (81.5, 181.5)
  line L768 (81.5, 181.5) -> (81.5, 198.5)
  line L769 (81.5, 198.5) -> (98.5, 198.5)
  line L770 (98.5, 198.5) -> (98.5, 181.5)
  line L771 (-81.5, 161.5) -> (-98.5, 161.5)
  line L772 (-98.5, 161.5) -> (-98.5, 178.5)
  line L773 (-98.5, 178.5) -> (-81.5, 178.5)
  line L774 (-81.5, 178.5) -> (-81.5, 161.5)
  line L775 (-61.5, 161.5) -> (-78.5, 161.5)
  line L776 (-78.5, 161.5) -> (-78.5, 178.5)
  line L777 (-78.5, 178.5) -> (-61.5, 178.5)
  line L778 (-61.5, 178.5) -> (-61.5, 161.5)
  line L779 (-41.5, 161.5) -> (-58.5, 161.5)
  line L780 (-58.5, 161.5) -> (-58.5, 178.5)
  line L781 (-58.5, 178.5) -> (-41.5, 178.5)
  line L782 (-41.5, 178.5) -> (-41.5, 161.5)
  line L783 (-21.5, 161.5) -> (-38.5, 161.5)
  line L784 (-38.5, 161.5) -> (-38.5, 178.5)
  line L785 (-38.5, 178.5) -> (-21.5, 178.5)
  line L786 (-21.5, 178.5) -> (-21.5, 161.5)
  line L787 (-1.5, 161.5) -> (-18.5, 161.5)
  line L788 (-18.5, 161.5) -> (-18.5, 178.5)
  line L789 (-18.5, 178.5) -> (-1.5, 178.5)
  line L790 (-1.5, 178.5) -> (-1.5, 161.5)
  line L791 (18.5, 161.5) -> (1.5, 161.5)
  line L792 (1.5, 161.5) -> (1.5, 178.5)
  line L793 (1.5, 178.5) -> (18.5, 178.5)
  line L794 (18.5, 178.5) -> (18.5, 161.5)
  line L795 (78.5, 121.5) -> (61.5, 121.5)
  line L796 (61.5, 121.5) -> (61.5, 138.5)
  line L797 (61.5, 138.5) -> (78.5, 138.5)
  line L798 (78.5, 138.5) -> (78.5, 121.5)
  line L799 (-21.5, -58.5) -> (-38.5, -58.5)
  line L800 (-38.5, -58.5) -> (-38.5, -41.5)
  line L801 (-38.5, -41.5) -> (-21.5, -41.5)
  line L802 (-21.5, -41.5) -> (-21.5, -58.5)
  line L803 (18.5, -58.5) -> (1.5, -58.5)
  line L804 (1.5, -58.5) -> (1.5, -41.5)
  line L805 (1.5, -41.5) -> (18.5, -41.5)
  line L806 (18.5, -41.5) -> (18.5, -58.5)
  line L807 (38.5, -58.5) -> (21.5, -58.5)
  line L808 (21.5, -58.5) -> (21.5, -41.5)
  line L809 (21.5, -41.5) -> (38.5, -41.5)
  line L810 (38.5, -41.5) -> (38.5, -58.5)
  line L811 (58.5, -58.5) -> (41.5, -58.5)
  line L812 (41.5, -58.5) -> (41.5, -41.5)
  line L813 (41.5, -41.5) -> (58.5, -41.5)
  line L814 (58.5, -41.5) -> (58.5, -58.5)
  line L815 (78.5, -58.5) -> (61.5, -58.5)
  line L816 (61.5, -58.5) -> (61.5, -41.5)
  line L817 (61.5, -41.5) -> (78.5, -41.5)
  line L818 (78.5, -41.5) -> (78.5, -58.5)
  line L819 (98.5, -58.5) -> (81.5, -58.5)
  line L820 (81.5, -58.5) -> (81.5, -41.5)
  line L821 (81.5, -41.5) -> (98.5, -41.5)
  line L822 (98.5, -41.5) -> (98.5, -58.5)
  line L823 (-81.5, -78.5) -> (-98.5, -78.5)
  line L824 (-98.5, -78.5) -> (-98.5, -61.5)
  line L825 (-98.5, -61.5) -> (-81.5, -61.5)
  line L826 (-81.5, -61.5) -> (-81.5, -78.5)
  line L827 (-61.5, -78.5) -> (-78.5, -78.5)
  line L828 (-78.5, -78.5) -> (-78.5, -61.5)
  line L829 (-78.5, -61.5) -> (-61.5, -61.5)
  line L830 (-61.5, -61.5) -> (-61.5, -78.5)
  line L831 (-41.5, -78.5) -> (-58.5, -78.5)
  line L832 (-58.5, -78.5) -> (-58.5, -61.5)
  line L833 (-58.5, -61.5) -> (-41.5, -61.5)
  line L834 (-41.5, -61.5) -> (-41.5, -78.5)
  line L835 (-21.5, -78.5) -> (-38.5, -78.5)
  line L836 (-38.5, -78.5) -> (-38.5, -61.5)
  line L837 (-38.5, -61.5) -> (-21.5, -61.5)
  line L838 (-21.5, -61.5) -> (-21.5, -78.5)
  line L839 (-1.5, -78.5) -> (-18.5, -78.5)
  line L840 (-18.5, -78.5) -> (-18.5, -61.5)
  line L841 (-18.5, -61.5) -> (-1.5, -61.5)
  line L842 (-1.5, -61.5) -> (-1.5, -78.5)
  line L843 (18.5, -78.5) -> (1.5, -78.5)
  line L844 (1.5, -78.5) -> (1.5, -61.5)
  line L845 (1.5, -61.5) -> (18.5, -61.5)
  line L846 (18.5, -61.5) -> (18.5, -78.5)
  line L847 (38.5, -78.5) -> (21.5, -78.5)
  line L848 (21.5, -78.5) -> (21.5, -61.5)
  line L849 (21.5, -61.5) -> (38.5, -61.5)
  line L850 (38.5, -61.5) -> (38.5, -78.5)
  line L851 (58.5, -78.5) -> (41.5, -78.5)
  line L852 (41.5, -78.5) -> (41.5, -61.5)
  line L853 (41.5, -61.5) -> (58.5, -61.5)
  line L854 (58.5, -61.5) -> (58.5, -78.5)
  line L855 (78.5, -78.5) -> (61.5, -78.5)
  line L856 (61.5, -78.5) -> (61.5, -61.5)
  line L857 (61.5, -61.5) -> (78.5, -61.5)
  line L858 (78.5, -61.5) -> (78.5, -78.5)
  line L859 (98.5, -78.5) -> (81.5, -78.5)
  line L860 (81.5, -78.5) -> (81.5, -61.5)
  line L861 (81.5, -61.5) -> (98.5, -61.5)
  line L862 (98.5, -61.5) -> (98.5, -78.5)
  line L863 (-81.5, -98.5) -> (-98.5, -98.5)
  line L864 (-98.5, -98.5) -> (-98.5, -81.5)
  line L865 (-98.5, -81.5) -> (-81.5, -81.5)
  line L866 (-81.5, -81.5) -> (-81.5, -98.5)
  line L867 (-61.5, -98.5) -> (-78.5, -98.5)
  line L868 (-78.5, -98.5) -> (-78.5, -81.5)
  line L869 (-78.5, -81.5) -> (-61.5, -81.5)
  line L870 (-61.5, -81.5) -> (-61.5, -98.5)
  line L871 (-41.5, -98.5) -> (-58.5, -98.5)
  line L872 (-58.5, -98.5) -> (-58.5, -81.5)
  line L873 (-58.5, -81.5) -> (-41.5, -81.5)
  line L874 (-41.5, -81.5) -> (-41.5, -98.5)
  line L875 (-21.5, -98.5) -> (-38.5, -98.5)
  line L876 (-38.5, -98.5) -> (-38.5, -81.5)
  line L877 (-38.5, -81.5) -> (-21.5, -81.5)
  line L878 (-21.5, -81.5) -> (-21.5, -98.5)
  line L879 (-1.5, -98.5) -> (-18.5, -98.5)
  line L880 (-18.5, -98.5) -> (-18.5, -81.5)
  line L881 (-18.5, -81.5) -> (-1.5, -81.5)
  line L882 (-1.5, -81.5) -> (-1.5, -98.5)
  line L883 (18.5, -98.5) -> (1.5, -98.5)
  line L884 (1.5, -98.5) -> (1.5, -81.5)
  line L885 (1.5, -81.5) -> (18.5, -81.5)
  line L886 (18.5, -81.5) -> (18.5, -98.5)
  line L887 (38.5, -98.5) -> (21.5, -98.5)
  line L888 (21.5, -98.5) -> (21.5, -81.5)
  line L889 (21.5, -81.5) -> (38.5, -81.5)
  line L890 (38.5, -81.5) -> (38.5, -98.5)
  line L891 (58.5, -98.5) -> (41.5, -98.5)
  line L892 (41.5, -98.5) -> (41.5, -81.5)
  line L893 (41.5, -81.5) -> (58.5, -81.5)
  line L894 (58.5, -81.5) -> (58.5, -98.5)
  line L895 (100, -220) -> (100, -200) construction
  circle A11 centre (100, -200) radius 2
  circle A12 centre (100, -160) radius 2
  circle A13 centre (100, -120) radius 2
  circle A14 centre (100, -80) radius 2
  circle A15 centre (100, -40) radius 2
  circle A16 centre (100, 0) radius 2
  circle A17 centre (100, 40) radius 2
  circle A18 centre (100, 80) radius 2
  circle A19 centre (100, 120) radius 2
  circle A20 centre (100, 160) radius 2
  circle A21 centre (100, 200) radius 2
  dimension "d28" = 20
  dimension "d29" = 4
  dimension "d32" = 400
  dimension "d33" = 0
  constraint coincident L11.end L12.start
  constraint perpendicular L11 L895
  constraint coincident L895.end A11.centre
  measures "d28" distance of L11.end L895.end
  measures "d29" diameter of A11
extrude "Extrude6" add sketch "Sketch4" along normal blind 1.6 contours L12 A21 | L12 A20 | L12 A19 | L12 A18 | L12 A17 | L12 A16 | L12 A15 | L12 A14 | L12 A13 | L12 A12 | L12 A11 picked at (99.8035, 200.637) picked at (99.8035, 160.637) picked at (99.5142, 119.3697) picked at (99.5142, 79.3697) picked at (99.7107, 39.3994) picked at (98.5211, 0.0862) picked at (99.7107, -40.6006) picked at (99.5142, -80.6303) picked at (99.5142, -120.6303) picked at (99.8035, -159.363) picked at (99.0858, -200.4157) bodies 1
sketch "Sketch5" plane through (0, 0, -1.6) normal (0, 0, -1) x (-1, 0, 0)
  line L0 (-105, 220) -> (-105, -220)
  line L1 (-105, -220) -> (-100, -220)
  line L2 (-100, -220) -> (-100, -202)
  arc A0 (-100, -202) -> (-100, -198) centre (-100, -200) ccw
  line L3 (-100, -198) -> (-100, -162)
  arc A1 (-100, -162) -> (-100, -158) centre (-100, -160) ccw
  line L4 (-100, -158) -> (-100, -122)
  arc A2 (-100, -122) -> (-100, -118) centre (-100, -120) ccw
  line L5 (-100, -118) -> (-100, -82)
  arc A3 (-100, -82) -> (-100, -78) centre (-100, -80) ccw
  line L6 (-100, -78) -> (-100, -42)
  arc A4 (-100, -42) -> (-100, -38) centre (-100, -40) ccw
  line L7 (-100, -38) -> (-100, -2)
  arc A5 (-100, -2) -> (-100, 2) centre (-100, 0) ccw
  line L8 (-100, 2) -> (-100, 38)
  arc A6 (-100, 38) -> (-100, 42) centre (-100, 40) ccw
  line L9 (-100, 42) -> (-100, 78)
  arc A7 (-100, 78) -> (-100, 82) centre (-100, 80) ccw
  line L10 (-100, 82) -> (-100, 118)
  arc A8 (-100, 118) -> (-100, 122) centre (-100, 120) ccw
  line L11 (-100, 122) -> (-100, 158)
  arc A9 (-100, 158) -> (-100, 162) centre (-100, 160) ccw
  line L12 (-100, 162) -> (-100, 198)
  arc A10 (-100, 198) -> (-100, 202) centre (-100, 200) ccw
  line L13 (-100, 202) -> (-100, 220)
  line L14 (-100, 220) -> (-105, 220)
  line L15 (-100, 200) -> (-105, 200)
  line L16 (-102.5, 200) -> (-100, 200)
  circle A11 centre (-101.25, 200) radius 3.175
  line L17 (-100, 120) -> (-105, 120)
  line L18 (-102.5, 120) -> (-100, 120)
  circle A12 centre (-101.25, 120) radius 3.175
  line L19 (-100, 40) -> (-105, 40)
  line L20 (-102.5, 40) -> (-100, 40)
  circle A13 centre (-101.25, 40) radius 3.175
  line L21 (-100, -40) -> (-105, -40)
  line L22 (-102.5, -40) -> (-100, -40)
  circle A14 centre (-101.25, -40) radius 3.175
  line L23 (-100, -120) -> (-105, -120)
  line L24 (-102.5, -120) -> (-100, -120)
  circle A15 centre (-101.25, -120) radius 3.175
  line L25 (-100, -200) -> (-105, -200)
  line L26 (-102.5, -200) -> (-100, -200)
  circle A16 centre (-101.25, -200) radius 3.175
  dimension "d36" = 6.35
  dimension "d37" = 6.35
  dimension "d38" = 6.35
  dimension "d39" = 6.35
  dimension "d40" = 6.35
  dimension "d41" = 6.35
  constraint coincident A10.centre L15.start
  constraint coincident L0 L15.end
  constraint perpendicular L0 L15
  constraint midpoint L15 L16.start
  constraint midpoint L16 A11.centre
  constraint coincident A8.centre L17.start
  constraint coincident L0 L17.end
  constraint perpendicular L0 L17
  constraint midpoint L17 L18.start
  constraint midpoint L18 A12.centre
  constraint coincident A6.centre L19.start
  constraint coincident L0 L19.end
  constraint perpendicular L0 L19
  constraint midpoint L19 L20.start
  constraint midpoint L20 A13.centre
  constraint coincident A4.centre L21.start
  constraint coincident L0 L21.end
  constraint perpendicular L0 L21
  constraint midpoint L21 L22.start
  constraint midpoint L22 A14.centre
  constraint coincident A2.centre L23.start
  constraint coincident L0 L23.end
  constraint perpendicular L0 L23
  constraint midpoint L23 L24.start
  constraint midpoint L24 A15.centre
  constraint coincident A0.centre L25.start
  constraint coincident L0 L25.end
  constraint perpendicular L0 L25
  constraint midpoint L25 L26.start
  constraint midpoint L26 A16.centre
  measures "d36" diameter of A11
  measures "d37" diameter of A12
  measures "d38" diameter of A13
  measures "d39" diameter of A14
  measures "d40" diameter of A15
  measures "d41" diameter of A16
extrude "Extrude7" add sketch "Sketch5" along normal blind 1.5875 contours L0 L13 L14 L15 A11 | L0 L11 A9 L12 L15 A11 L17 A12 | L0 L9 A7 L10 L17 A12 L19 A13 | L0 L7 A5 L8 L19 A13 L21 A14 | L0 L5 A3 L6 L21 A14 L23 A15 | L0 L3 A1 L4 L23 A15 L25 A16 | L0 L1 L2 L25 A16 bodies 1
sketch "Sketch6" plane through (0, 0, -1.6) normal (0, 0, -1) x (-1, 0, 0)
  line L0 (100, 220) -> (100, 202)
  arc A0 (100, 202) -> (100, 198) centre (100, 200) ccw
  line L1 (100, 198) -> (100, 162)
  arc A1 (100, 162) -> (100, 158) centre (100, 160) ccw
  line L2 (100, 158) -> (100, 122)
  arc A2 (100, 122) -> (100, 118) centre (100, 120) ccw
  line L3 (100, 118) -> (100, 82)
  arc A3 (100, 82) -> (100, 78) centre (100, 80) ccw
  line L4 (100, 78) -> (100, 42)
  arc A4 (100, 42) -> (100, 38) centre (100, 40) ccw
  line L5 (100, 38) -> (100, 2)
  arc A5 (100, 2) -> (100, -2) centre (100, 0) ccw
  line L6 (100, -2) -> (100, -38)
  arc A6 (100, -38) -> (100, -42) centre (100, -40) ccw
  line L7 (100, -42) -> (100, -78)
  arc A7 (100, -78) -> (100, -82) centre (100, -80) ccw
  line L8 (100, -82) -> (100, -118)
  arc A8 (100, -118) -> (100, -122) centre (100, -120) ccw
  line L9 (100, -122) -> (100, -158)
  arc A9 (100, -158) -> (100, -162) centre (100, -160) ccw
  line L10 (100, -162) -> (100, -198)
  arc A10 (100, -198) -> (100, -202) centre (100, -200) ccw
  line L11 (100, -202) -> (100, -220)
  line L12 (100, -220) -> (105, -220)
  line L13 (105, -220) -> (105, 220)
  line L14 (105, 220) -> (100, 220)
  line L15 (100, 200) -> (105, 200)
  line L16 (102.5, 200) -> (100, 200)
  circle A11 centre (101.25, 200) radius 3.175
  line L17 (100, 120) -> (105, 120)
  line L18 (102.5, 120) -> (100, 120)
  circle A12 centre (101.25, 120) radius 3.175
  line L19 (100, 40) -> (105, 40)
  line L20 (102.5, 40) -> (100, 40)
  circle A13 centre (101.25, 40) radius 3.175
  line L21 (100, -40) -> (105, -40)
  line L22 (102.5, -40) -> (100, -40)
  circle A14 centre (101.25, -40) radius 3.175
  line L23 (100, -120) -> (105, -120)
  line L24 (102.5, -120) -> (100, -120)
  circle A15 centre (101.25, -120) radius 3.175
  line L25 (100, -200) -> (105, -200)
  line L26 (102.5, -200) -> (100, -200)
  circle A16 centre (101.25, -200) radius 3.175
  dimension "d44" = 6.35
  dimension "d45" = 6.35
  dimension "d46" = 6.35
  dimension "d47" = 6.35
  dimension "d48" = 6.35
  dimension "d49" = 6.35
  constraint coincident A0.centre L15.start
  constraint coincident L13 L15.end
  constraint perpendicular L13 L15
  constraint midpoint L15 L16.start
  constraint midpoint L16 A11.centre
  constraint coincident A2.centre L17.start
  constraint coincident L13 L17.end
  constraint perpendicular L13 L17
  constraint midpoint L17 L18.start
  constraint midpoint L18 A12.centre
  constraint coincident A4.centre L19.start
  constraint coincident L13 L19.end
  constraint perpendicular L13 L19
  constraint midpoint L19 L20.start
  constraint midpoint L20 A13.centre
  constraint coincident A6.centre L21.start
  constraint coincident L13 L21.end
  constraint perpendicular L13 L21
  constraint midpoint L21 L22.start
  constraint midpoint L22 A14.centre
  constraint coincident A8.centre L23.start
  constraint coincident L13 L23.end
  constraint perpendicular L13 L23
  constraint midpoint L23 L24.start
  constraint midpoint L24 A15.centre
  constraint coincident A10.centre L25.start
  constraint coincident L13 L25.end
  constraint perpendicular L13 L25
  constraint midpoint L25 L26.start
  constraint midpoint L26 A16.centre
  measures "d44" diameter of A11
  measures "d45" diameter of A12
  measures "d46" diameter of A13
  measures "d47" diameter of A14
  measures "d48" diameter of A15
  measures "d49" diameter of A16
extrude "Extrude8" add sketch "Sketch6" along normal blind 1.5875 contours L0 L13 L14 L15 A11 | L1 A1 L2 L13 L15 A11 L17 A12 | L3 A3 L4 L13 L17 A12 L19 A13 | L5 A5 L6 L13 L19 A13 L21 A14 | L7 A7 L8 L13 L21 A14 L23 A15 | L9 A9 L10 L13 L23 A15 L25 A16 | L11 L12 L13 L25 A16 bodies 1
extrude "Extrude9" add 1 faces at (-102.8333, 26.1667, 13) along direction (0, 0, 1) blind 3 separate body on bodies 1 makes body 2